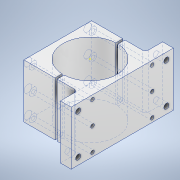
# Autodesk Inventor part: Spindel100mm
Saved by Autodesk Inventor 2020.1 (Build 241239000, 239)
## iProperties
Created: 2023-01-15
Part Number: Spindel100mm
Material: Алюминий 6061
Document SubType Name: Modeling
Designer: KirikDK
Density: 2.7 g/cm^3
Appearance: Алюминий — плоский
Mass: 2199.42 g
Surface Area: 1097.08 cm^2
Volume: 814.602 cm^3
Author: KirikDK
Autodesk Inventor part; units mm, degrees
ref_plane "YZ Plane" through (0, 0, 0) normal (1, 0, 0) x (0, 1, 0)
ref_plane "XZ Plane" through (0, 0, 0) normal (0, 1, 0) x (-1, 0, 0)
ref_plane "XY Plane" through (0, 0, 0) normal (0, 0, 1) x (1, 0, 0)
sketch "Эскиз1" plane through (0, 0, 0) normal (0, 1, 0) x (-1, 0, 0)
  circle A0 centre (0, 0) radius 50
  line L0 (60, 63) -> (-60, 63)
  line L1 (-60, 63) -> (-60, -63)
  line L2 (-60, -63) -> (60, -63)
  line L3 (60, -63) -> (60, 63)
  line L4 (-60, -63) -> (-40, -63)
  line L5 (-40, -63) -> (-40, -95)
  line L6 (-40, -95) -> (-60, -95)
  line L7 (-60, -95) -> (-60, -63)
  line L8 (-60, 63) -> (-40, 63)
  line L9 (-40, 63) -> (-40, 95)
  line L10 (-40, 95) -> (-60, 95)
  line L11 (-60, 95) -> (-60, 63)
  point P0 (-40, 63)
  dimension "d0" = 100
  dimension "d1" = 32
  dimension "d2" = 32
  dimension "d3" = 20
  dimension "d4" = 20
  dimension "d5" = 120
  dimension "d6" = 126
  dimension "d7" = 63
  dimension "d8" = 63
  constraints: 24 end point, 6 parallel, 3 horizontal, 3 perpendicular, 1 centre point, 1 coincident, 1 point on line
  measures "d0" diameter of A0
  measures "d1" distance between parallel lines of L0 L10
  measures "d2" distance between parallel lines of L6 L2
  measures "d3" distance between parallel lines of L5 L7
  measures "d4" distance between parallel lines of L9 L11
  measures "d5" distance between parallel lines of L3 L1
  measures "d6" distance between parallel lines of L0 L2
  measures "d7" distance from line of point (0, 0) L2
  measures "d8" distance from line of point (0, 0) L0
extrude "Выдавливание1" add sketch "Эскиз1" along normal blind 100
sketch "Эскиз2" plane through (0, 100, 0) normal (0, 1, 0) x (1, 0, 0)
  point P0 (0, 0)
fillet "Сопряжение1" radius 6 2 edges at (40, 50, 63) (40, 50, -63)
sketch "Эскиз3" plane through (40, 0, 95) normal (-1, 0, 0) x (0, 0, 1)
  line L0 (-164, 100) -> (-164, 0) projected
  line L1 (-190, 100) -> (-164, 100) projected
  line L2 (-190, 0) -> (-190, 100) projected
  line L3 (-190, 0) -> (-164, 0) projected
  line L4 (-26, 0) -> (-26, 100) projected
  line L5 (-26, 0) -> (0, 0) projected
  line L6 (0, 0) -> (0, 100) projected
  line L7 (-26, 100) -> (0, 100) projected
  line L8 (-177, 87) -> (-177, 87)
  line L9 (-177, 87) -> (-177, 13)
  line L10 (-177, 13) -> (-177, 13)
  line L11 (-177, 13) -> (-177, 87)
  line L12 (-13, 87) -> (-13, 13)
  line L13 (-13, 13) -> (-13, 13)
  line L14 (-13, 13) -> (-13, 87)
  line L15 (-13, 87) -> (-13, 87)
  circle A0 centre (-13, 87) radius 4.75
  circle A1 centre (-13, 13) radius 4.75
  circle A2 centre (-177, 87) radius 4.75
  circle A3 centre (-177, 13) radius 4.75
  point P0 (-95, 0)
  dimension "d12" = 13
  dimension "d13" = 13
  constraints: 16 end point, 4 centre point, 4 coincident, 6 other
  measures "d12" distance between parallel lines of L2 L11
  measures "d13" distance between parallel lines of L12 L6
extrude "Выдавливание2" cut sketch "Эскиз3" against normal blind 25 contours A3 | A2 | A1 | A0
sketch "Эскиз4" plane through (-60, 0, -63) normal (-1, 0, 0) x (0, 0, 1)
  line L0 (0, 0) -> (126, 0) projected
  line L1 (126, 0) -> (126, 100) projected
  line L2 (0, 100) -> (126, 100) projected
  line L3 (0, 0) -> (0, 100) projected
  line L4 (7.5, 92.5) -> (118.5, 92.5)
  line L5 (118.5, 92.5) -> (118.5, 7.5)
  line L6 (118.5, 7.5) -> (7.5, 7.5)
  line L7 (7.5, 7.5) -> (7.5, 92.5)
  circle A0 centre (7.5, 7.5) radius 3.5
  circle A1 centre (7.5, 92.5) radius 3.5
  circle A2 centre (118.5, 92.5) radius 3.5
  circle A3 centre (118.5, 7.5) radius 3.5
  circle A4 centre (118.5, 50) radius 3.5
  circle A5 centre (7.5, 50) radius 3.5
  point P0 (63, 0)
  dimension "d16" = 7.5
  constraints: 8 end point, 6 centre point, 4 coincident, 2 midpoint, 3 other
  measures "d16" distance between parallel lines of L3 L7
hole "Отверстие1" at (-60, 7.5, -55.5) at (-60, 50, -55.5) at (-60, 92.5, -55.5) at (-60, 92.5, 55.5) at (-60, 50, 55.5) at (-60, 7.5, 55.5) direction (1, 0, 0) diameter 6.7 end through all counterbore diameter 14 counterbore depth 10
sketch "Эскиз5" plane through (0, 100, 0) normal (0, 1, 0) x (1, 0, 0)
  line L0 (-2, -66) -> (2, -66)
  line L1 (2, -66) -> (2, 67)
  line L2 (2, 67) -> (-2, 67)
  line L3 (-2, 67) -> (-2, -66)
  point P0 (0, 0)
  constraints: 8 end point, 2 parallel, 1 horizontal, 1 perpendicular
extrude "Выдавливание3" cut sketch "Эскиз5" against normal blind 200
